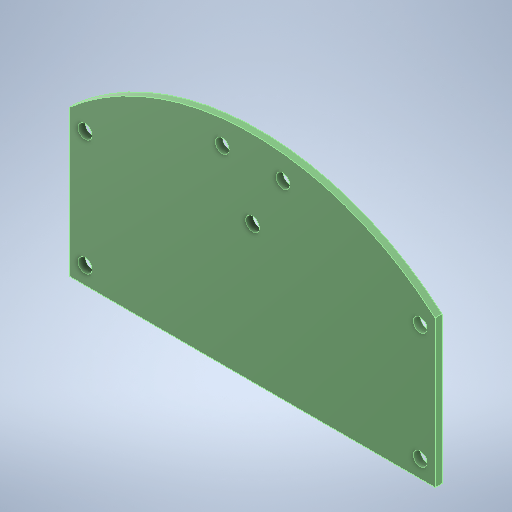
# Autodesk Inventor part: SensorBoard-SPG27
Saved by Autodesk Inventor 2025.3 (Build 293356030, 356C)
## iProperties
Created: 2025-05-29
Part Number: SensorBoard-SPG27
Material: 一般
Document SubType Name: Modeling
Designer: yamashita1
Density: 1 g/cm^3
Appearance: 滑らか - 濃い深緑
Author: yamashita1
Autodesk Inventor part; units mm, degrees
ref_plane "YZ Plane" through (0, 0, 0) normal (1, 0, 0) x (0, 1, 0)
ref_plane "XZ Plane" through (0, 0, 0) normal (0, 1, 0) x (-1, 0, 0)
ref_plane "XY Plane" through (0, 0, 0) normal (0, 0, 1) x (1, 0, 0)
sketch "スケッチ1" plane through (0, 0, 0) normal (0, 0, 1) x (1, 0, 0)
  circle A0 centre (0, 0) radius 65 construction
  line L0 (-42.5, 65) -> (42.5, 65) construction
  line L1 (42.5, 65) -> (42.5, -65) construction
  line L2 (42.5, -65) -> (-42.5, -65) construction
  line L3 (-42.5, -65) -> (-42.5, 65) construction
  arc A1 (42.5, 49.1808) -> (-42.5, 49.1808) centre (0, 0) ccw
  line L4 (-42.5, 49.1808) -> (-42.5, -49.1808)
  line L5 (42.5, 49.1808) -> (42.5, -49.1808)
  arc A2 (-42.5, -49.1808) -> (42.5, -49.1808) centre (0, 0) ccw
  line L6 (42.5, -49) -> (-42.5, -49)
  line L7 (-42.5, 15) -> (42.5, 15)
  point P0 (0, 65)
  dimension "d0" = 130
  dimension "d1" = 85
  dimension "d41" = 49
  dimension "d52" = 15
  constraints: 18 end point, 9 point on circle, 8 point on line, 3 centre point, 3 parallel, 3 perpendicular, 2 tangent, 1 coincident, 1 concentric, 1 horizontal, 1 midpoint, 1 vertical, 1 vertical alignment
  measures "d0" diameter of A0
  measures "d1" distance of L1.end L2.end
  measures "d41" distance from line of point (0, 0) L6
  measures "d52" distance from line of L7 point (0, 0)
extrude "基板" add sketch "スケッチ1" along normal blind 1.6 contours L5 L7 L4 A1
sketch "スケッチ3" plane through (0, 0, 1.6) normal (0, 0, 1) x (1, 0, 0)
  line L0 (0, 0) -> (0, 55.332) construction
  line L1 (-15.38, 55) -> (15.38, 55) construction
  line L2 (0, 46.85) -> (-7.0581, 50.925) construction
  line L3 (-7.0581, 50.925) -> (-7.0581, 59.075) construction
  line L4 (-7.0581, 59.075) -> (0, 63.15) construction
  line L5 (0, 63.15) -> (7.0581, 59.075) construction
  line L6 (7.0581, 59.075) -> (7.0581, 50.925) construction
  line L7 (7.0581, 50.925) -> (0, 46.85) construction
  arc A0 (42.5, 49.1808) -> (-42.5, 49.1808) centre (0, 0) ccw construction
  point P0 (0, 55)
  point P1 (0, 55)
  point P2 (0, 65)
  dimension "d17" = 16.3
  dimension "d18" = 10
  constraints: 16 end point, 7 coincident, 2 point on line, 1 horizontal, 1 midpoint, 1 point on circle, 1 vertical, 13 other
  measures "d17" distance of L2.start L4.end
  measures "d18" distance from line of point (0, 65) L1
hole "ボールキャスター取付穴" at (-7.0581, 59.075, 1.6) at (7.0581, 59.075, 1.6) at (0, 46.85, 1.6) direction (0, 0, -1) diameter 3.2 end through all
sketch "スケッチ5" plane through (0, 0, 1.6) normal (0, 0, 1) x (1, 0, 0)
  line L0 (0, 0) -> (0, 96.0936) construction
  line L1 (-67.6385, -10) -> (77.8935, -10) construction
  point P0 (-39, 46)
  point P1 (39, 46)
  point P2 (-39, 19)
  point P3 (39, 19)
  dimension "d42" = 78
  dimension "d43" = 10
  dimension "d44" = 56
  dimension "d53" = 27
  constraints: 4 end point, 2 horizontal alignment, 2 vertical alignment, 1 horizontal, 1 symmetric about line, 1 vertical
  measures "d42" distance of point (39, 46) point (-39, 46)
  measures "d43" distance from line of L1 L0.start
  measures "d44" distance from line of point (39, 46) L1
  measures "d53" distance of point (-39, 19) point (-39, 46)
hole "連結穴" at (-39, 46, 1.6) at (39, 46, 1.6) at (-39, 19, 1.6) at (39, 19, 1.6) direction (0, 0, -1) diameter 3.2 end through all
